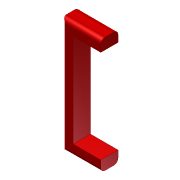
# Autodesk Inventor part: Bumpers_Red
Saved by Autodesk Inventor 2012 (Build 160160000, 160)
## iProperties
Created: 2012-02-26
Part Number: Bumpers_Red
Material: Default
Document SubType Name: Modeling
Designer: JesseK
Surface Area: 5076.99 cm^2
Volume: 12578.2 cm^3
Author: JesseK
Autodesk Inventor part; units mm, degrees
ref_plane "YZ Plane" through (0, 0, 0) normal (1, 0, 0) x (0, 1, 0)
ref_plane "XZ Plane" through (0, 0, 0) normal (0, 1, 0) x (-1, 0, 0)
ref_plane "XY Plane" through (0, 0, 0) normal (0, 0, 1) x (1, 0, 0)
sketch "Sketch1" plane through (0, 0, 0) normal (0, 0, 1) x (1, 0, 0)
  line L0 (0, 0) -> (285.75, 0)
  line L1 (285.75, 850.9) -> (0, 850.9)
  line L2 (0, 850.9) -> (0, 0)
  line L3 (285.75, 768.35) -> (82.55, 768.35)
  line L4 (82.55, 768.35) -> (82.55, 82.55)
  line L5 (82.55, 82.55) -> (285.75, 82.55)
  line L6 (285.75, 0) -> (285.75, 82.55)
  line L7 (285.75, 768.35) -> (285.75, 850.9)
  dimension "d0" = 82.55
  dimension "d1" = 82.55
  dimension "d3" = 203.2
  dimension "d4" = 203.2
  dimension "d5" = 685.8
  dimension "d6" = 82.55
  constraints: 16 end point, 4 parallel, 3 perpendicular, 2 horizontal
  measures "d0" distance of L3.start L1.start
  measures "d1" distance of L0.end L5.end
  measures "d3" distance of L3.start L3.end
  measures "d4" distance of L4.end L5.end
  measures "d5" distance of L3.end L4.end
  measures "d6" distance between parallel lines of L2 L4
extrude "Extrusion1" add sketch "Sketch1" along normal blind 127
fillet "Fillet1" radius 31.75 6 edges at (142.875, 850.9, 127) (142.875, 850.9, 0) (0, 425.45, 127) (0, 425.45, 0) (142.875, 0, 127) (142.875, 0, 0)
body "Solid1"
